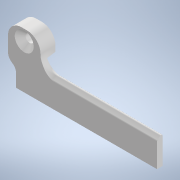
# Autodesk Inventor part: wifi_fixator
Saved by Autodesk Inventor 2022 (Build 260153000, 153)
## iProperties
Created: 2025-01-04
Part Number: wifi_fixator
Material: Типовые
Document SubType Name: Modeling
Designer: akap
Density: 1 g/cm^3
Appearance: По умолчанию
Author: akap
Autodesk Inventor part; units mm, degrees
ref_plane "YZ Plane" through (0, 0, 0) normal (1, 0, 0) x (0, 1, 0)
ref_plane "XZ Plane" through (0, 0, 0) normal (0, 1, 0) x (-1, 0, 0)
ref_plane "XY Plane" through (0, 0, 0) normal (0, 0, 1) x (1, 0, 0)
sketch "Эскиз1" plane through (0, 0, 0) normal (0, 0, 1) x (1, 0, 0)
  line L0 (26, -11.6) -> (-26, -11.6)
  line L1 (-26, -11.6) -> (-26, 11.6)
  line L2 (-26, 11.6) -> (26, 11.6)
  line L3 (26, 11.6) -> (26, -11.6)
  line L4 (-27, -1.6037) -> (27, -1.6037)
  line L5 (27, -8.6037) -> (27, -1.6037)
  line L6 (-27, -8.6037) -> (27, -8.6037)
  line L7 (-27, -1.6037) -> (-27, -8.6037)
  line L8 (-25.5, 7) -> (21, 7)
  arc A0 (23, 5) -> (21, 7) centre (21, 5) ccw
  line L9 (23, 5) -> (23, -5)
  arc A1 (21, -7) -> (23, -5) centre (21, -5) ccw
  line L10 (21, -7) -> (-29, -7)
  arc A2 (-31, -5) -> (-29, -7) centre (-29, -5) ccw
  line L11 (-31, -5) -> (-31, 5)
  arc A3 (-30, 6.7321) -> (-31, 5) centre (-29, 5) ccw
  circle A4 centre (-50, 0.4) radius 1.35
  circle A5 centre (50, 0.4) radius 1.35
  arc A6 (-33.5169, 9.4302) -> (-33.5169, 14.4302) centre (-33.5169, 11.9302) ccw
  line L12 (-33.5169, 9.4302) -> (-38.5969, 9.4302)
  arc A7 (-38.5969, 14.4302) -> (-38.5969, 9.4302) centre (-38.5969, 11.9302) ccw
  line L13 (-38.5969, 14.4302) -> (-33.5169, 14.4302)
  line L14 (-39.1, 22.9302) -> (-31.1, 22.9302)
  arc A8 (-30.1, 21.9302) -> (-31.1, 22.9302) centre (-31.1, 21.9302) ccw
  line L15 (-30.1, 21.9302) -> (-30.1, 18.9302)
  arc A9 (-31.1, 17.9302) -> (-30.1, 18.9302) centre (-31.1, 18.9302) ccw
  line L16 (-31.1, 17.9302) -> (-39.1, 17.9302)
  arc A10 (-40.1, 18.9302) -> (-39.1, 17.9302) centre (-39.1, 18.9302) ccw
  line L17 (-40.1, 18.9302) -> (-40.1, 21.9302)
  arc A11 (-39.1, 22.9302) -> (-40.1, 21.9302) centre (-39.1, 21.9302) ccw
  arc A12 (-8.8, 26.9302) -> (-6.8, 28.9302) centre (-8.8, 28.9302) ccw
  line L18 (-6.8, 28.9302) -> (-6.8, 33.6939)
  arc A13 (-3.8, 36.6939) -> (-6.8, 33.6939) centre (-3.8, 33.6939) ccw
  line L19 (-3.8, 36.6939) -> (15.7, 36.6939)
  arc A14 (18.7, 33.6939) -> (15.7, 36.6939) centre (15.7, 33.6939) ccw
  line L20 (18.7, 33.6939) -> (18.7, 19.9302)
  arc A15 (15.7, 16.9302) -> (18.7, 19.9302) centre (15.7, 19.9302) ccw
  line L21 (15.7, 16.9302) -> (-14.8, 16.9302)
  arc A16 (-16.8, 18.9302) -> (-14.8, 16.9302) centre (-14.8, 18.9302) ccw
  line L22 (-16.8, 18.9302) -> (-16.8, 24.9302)
  arc A17 (-14.8, 26.9302) -> (-16.8, 24.9302) centre (-14.8, 24.9302) ccw
  line L23 (-14.8, 26.9302) -> (-8.8, 26.9302)
  circle A18 centre (23.0046, 15.7286) radius 1.5
  circle A19 centre (-23.0046, 15.7286) radius 1.5
  line L24 (-21.9, 127.8) -> (-29.3, 127.8)
  line L25 (-29.3, 127.8) -> (-29.3, 142.3)
  line L26 (-29.3, 142.3) -> (-21.9, 142.3)
  line L27 (-21.9, 142.3) -> (-21.9, 127.8)
  line L28 (29.3, 127.8) -> (21.9, 127.8)
  line L29 (21.9, 127.8) -> (21.9, 142.3)
  line L30 (21.9, 142.3) -> (29.3, 142.3)
  line L31 (29.3, 142.3) -> (29.3, 127.8)
  line L32 (-17.5, 135.4) -> (-17.5, 146.4)
  line L33 (-52.7636, 146.4) -> (-17.5, 146.4)
  spline S0 degree 4 poles (-62.3095, 142.4) (-60.4837, 144.6746) (-58.1635, 146.0345) (-55.4517, 146.4) (-52.7636, 146.4) knots 0 0 0 0 0 1 1 1 1 1
  spline S1 degree 4 poles (-66.7947, 122.4) (-66.7947, 127.5863) (-66.4694, 134.187) (-64.879, 139.1991) (-62.3095, 142.4) knots 0 0 0 0 0 0.584588 0.584588 0.584588 0.584588 0.584588
  line L34 (-66.7947, 12.4) -> (-66.7947, 122.4)
  spline S2 degree 4 poles (-62.3095, -7.6) (-64.879, -4.3991) (-66.4694, 0.613) (-66.7947, 7.2137) (-66.7947, 12.4) knots 0.415412 0.415412 0.415412 0.415412 0.415412 1 1 1 1 1
  spline S3 degree 4 poles (-52.7636, -11.6) (-55.4517, -11.6) (-58.1635, -11.2345) (-60.4837, -9.8746) (-62.3095, -7.6) knots 0 0 0 0 0 1 1 1 1 1
  line L35 (52.7636, -11.6) -> (-52.7636, -11.6)
  spline S4 degree 4 poles (62.3095, -7.6) (60.4837, -9.8746) (58.1635, -11.2345) (55.4517, -11.6) (52.7636, -11.6) knots 0 0 0 0 0 1 1 1 1 1
  spline S5 degree 4 poles (66.7947, 12.4) (66.7947, 7.2137) (66.4694, 0.613) (64.879, -4.3991) (62.3095, -7.6) knots 0 0 0 0 0 0.584588 0.584588 0.584588 0.584588 0.584588
  line L36 (66.7947, 122.4) -> (66.7947, 12.4)
  spline S6 degree 4 poles (62.3095, 142.4) (64.879, 139.1991) (66.4694, 134.187) (66.7947, 127.5863) (66.7947, 122.4) knots 0.415412 0.415412 0.415412 0.415412 0.415412 1 1 1 1 1
  spline S7 degree 4 poles (52.7636, 146.4) (55.4517, 146.4) (58.1635, 146.0345) (60.4837, 144.6746) (62.3095, 142.4) knots 0 0 0 0 0 1 1 1 1 1
  line L37 (17.5, 146.4) -> (52.7636, 146.4)
  line L38 (17.5, 146.4) -> (17.5, 135.4)
  line L39 (17.5, 135.4) -> (6, 135.4)
  line L40 (6, 135.4) -> (6, 130.5467)
  arc A20 (5, 129.5467) -> (6, 130.5467) centre (5, 130.5467) ccw
  line L41 (5, 129.5467) -> (-5, 129.5467)
  arc A21 (-6, 130.5467) -> (-5, 129.5467) centre (-5, 130.5467) ccw
  line L42 (-6, 130.5467) -> (-6, 135.4)
  line L43 (-6, 135.4) -> (-17.5, 135.4)
  circle A22 centre (-25.5, 37.9) radius 1.25
  circle A23 centre (25.5, 96.9) radius 1.25
  circle A24 centre (-25.5, 96.9) radius 1.25
  circle A25 centre (25.5, 37.9) radius 1.25
  arc A26 (22.1, 92.345) -> (25.1, 89.345) centre (25.1, 92.345) ccw
  line L44 (25.1, 89.345) -> (43.5, 89.345)
  line L45 (43.5, 125.4) -> (43.5, 89.345)
  arc A27 (45.5, 127.4) -> (43.5, 125.4) centre (45.5, 125.4) ccw
  line L46 (45.5, 127.4) -> (60.7947, 127.4)
  arc A28 (62.7947, 125.4) -> (60.7947, 127.4) centre (60.7947, 125.4) ccw
  line L47 (62.7947, 125.4) -> (62.7947, 9.4)
  arc A29 (60.7947, 7.4) -> (62.7947, 9.4) centre (60.7947, 9.4) ccw
  line L48 (60.7947, 7.4) -> (45.5, 7.4)
  arc A30 (43.5, 9.4) -> (45.5, 7.4) centre (45.5, 9.4) ccw
  line L49 (43.5, 45.3296) -> (43.5, 9.4)
  line L50 (43.5, 45.3296) -> (27.6138, 45.3296)
  line L51 (27.6138, 45.3296) -> (27.6138, 44.2037)
  line L52 (27.6138, 44.2037) -> (10.238, 44.2037)
  line L53 (10.238, 44.2037) -> (10.238, 45.3296)
  line L54 (10.238, 45.3296) -> (5, 45.3296)
  line L55 (5, 45.3296) -> (5, 42.3296)
  line L56 (5, 42.3296) -> (-5, 42.3296)
  line L57 (-5, 42.3296) -> (-5, 45.3296)
  line L58 (-5, 45.3296) -> (-10.238, 45.3296)
  line L59 (-10.238, 45.3296) -> (-10.238, 44.2037)
  line L60 (-10.238, 44.2037) -> (-27.6138, 44.2037)
  line L61 (-27.6138, 44.2037) -> (-27.6138, 45.3296)
  line L62 (-27.6138, 45.3296) -> (-29.6, 45.3296)
  line L63 (-29.6, 45.3296) -> (-29.6, 27.7796)
  line L64 (-29.6, 27.7796) -> (-40.6, 27.7796)
  line L65 (-40.6, 27.7796) -> (-40.6, 45.3296)
  line L66 (-40.6, 45.3296) -> (-43.5, 45.3296)
  line L67 (-43.5, 9.4) -> (-43.5, 45.3296)
  arc A31 (-45.5, 7.4) -> (-43.5, 9.4) centre (-45.5, 9.4) ccw
  line L68 (-45.5, 7.4) -> (-60.7947, 7.4)
  arc A32 (-62.7947, 9.4) -> (-60.7947, 7.4) centre (-60.7947, 9.4) ccw
  line L69 (-62.7947, 9.4) -> (-62.7947, 125.4)
  arc A33 (-60.7947, 127.4) -> (-62.7947, 125.4) centre (-60.7947, 125.4) ccw
  line L70 (-60.7947, 127.4) -> (-45.5, 127.4)
  arc A34 (-43.5, 125.4) -> (-45.5, 127.4) centre (-45.5, 125.4) ccw
  line L71 (-43.5, 89.345) -> (-43.5, 125.4)
  line L72 (-43.5, 89.345) -> (-40.6, 89.345)
  line L73 (-40.6, 89.345) -> (-40.6, 104.345)
  line L74 (-40.6, 104.345) -> (-28.1, 104.345)
  line L75 (-28.1, 104.345) -> (-28.1, 89.345)
  line L76 (-28.1, 89.345) -> (-18.1, 89.345)
  arc A35 (-18.1, 89.345) -> (-15.1, 92.345) centre (-18.1, 92.345) ccw
  line L77 (-15.1, 92.345) -> (-15.1, 99.8467)
  arc A36 (-12.1, 102.8467) -> (-15.1, 99.8467) centre (-12.1, 99.8467) ccw
  line L78 (-12.1, 102.8467) -> (19.1, 102.8467)
  arc A37 (22.1, 99.8467) -> (19.1, 102.8467) centre (19.1, 99.8467) ccw
  line L79 (22.1, 99.8467) -> (22.1, 92.345)
  line L80 (28, -0.6037) -> (-28, -0.6037)
  line L81 (-28, -0.6037) -> (-28, -9.6037)
  line L82 (-28, -9.6037) -> (28, -9.6037)
  line L83 (28, -9.6037) -> (28, -0.6037)
  line L84 (-40.5, 5.2533) -> (-27, 5.2533)
  line L85 (-27, 5.2533) -> (-27, -1.6037)
  line L86 (-26, -1.6037) -> (-26, 6.2533)
  line L87 (-26, 6.2533) -> (-40.5, 6.2533)
  line L88 (-26, 6.2533) -> (-29, 6.2533)
  line L89 (-29, 6.2533) -> (-29, 19.7286)
  line L90 (-29, 19.7286) -> (-17, 19.7286)
  line L91 (-17, 19.7286) -> (-17, 7)
  line L92 (-26, -1.6037) -> (27, -1.6037)
  line L93 (27, -1.6037) -> (27, 7)
  line L94 (27, 7) -> (-26, 7)
  line L95 (-26, 7) -> (-26, -1.6037)
  arc A38 (-30, 6.7321) -> (-29.5, 7.5981) centre (-30.5, 7.5981) ccw
  line L96 (-29.5, 7.5981) -> (-29.5, 12.6)
  line L97 (-29.5, 12.6) -> (-26.5, 12.6)
  line L98 (-26.5, 12.6) -> (-26.5, 8)
  arc A39 (-26.5, 8) -> (-25.5, 7) centre (-25.5, 8) ccw
  point P0 (0, 0)
  point P1 (26, -0.6037)
  point P2 (-17, 11.6)
  point P3 (-29, 7)
  point P4 (-26, 7)
  point P5 (-26, -0.6037)
  point P6 (23, -0.6037)
  point P7 (-26, -7)
  point P8 (-29, 12.6)
  point P9 (-26, 7.134)
  dimension "d0" = 1
  dimension "d1" = 1
  dimension "d2" = 3
  dimension "d3" = 4
  dimension "d4" = 12
  constraints: 28 end point, 3 collinear, 3 perpendicular, 2 parallel, 2 point on line, 1 horizontal, 1 vertical, 4 other
  measures "d0" distance between parallel lines of L4 L80
  measures "d1" distance between parallel lines of L85 L86
  measures "d2" distance of L86.end L88.end
  measures "d3" distance from line of L90 A19.centre
  measures "d4" distance between parallel lines of L89 L91
extrude "Выдавливание1" add sketch "Эскиз1" along normal blind 2 contours L80 L9 A0 L94 L3 | L94 L8 L91 L2 L3 | L80 L1 L94 L8 A0 L9 | L87 L89 L97 L98 A39 L1 | L91 L8 A39 L1 L2 | L2 L1 A39 L98 L97 L89 L90 L91 | L1 A39 L94
sketch "Эскиз2" plane through (0, 0, 0) normal (0, 0, -1) x (-1, 0, 0)
  line L0 (-26, -0.6037) -> (-26, 11.6) projected
  line L1 (-26, 11.6) -> (17, 11.6) projected
  line L2 (17, 11.6) -> (17, 19.7286) projected
  line L3 (17, 19.7286) -> (29, 19.7286) projected
  line L4 (29, 19.7286) -> (29, 6.2533) projected
  line L5 (26, 6.2533) -> (26, -0.6037) projected
  line L6 (26, -0.6037) -> (-26, -0.6037) projected
  line L7 (-26, -11.6) -> (26, -11.6) projected
  line L8 (-26, 11.6) -> (-26, -11.6) projected
  line L9 (26, 11.6) -> (-26, 11.6) projected
  line L10 (26, -11.6) -> (26, 11.6) projected
  line L11 (-27, 12.6) -> (-27, -12.6)
  line L12 (-27, -12.6) -> (27, -12.6)
  line L13 (27, -12.6) -> (27, 12.6)
  line L14 (27, 12.6) -> (-27, 12.6)
  line L15 (29, 6.2533) -> (26, 6.2533) projected
  circle A0 centre (23.0046, 15.7286) radius 1.5 projected
  point P0 (0, 0)
  point P1 (26, 7)
  point P2 (17, 12.6)
  point P3 (27, 6.2533)
  dimension "d7" = 1
  constraints: 8 end point, 3 other
  measures "d7" distance between parallel lines of L9 L14
extrude "Выдавливание2" add sketch "Эскиз2" along normal blind 3.5 contours L2 L3 L4 L15 L13 L14
fillet "Сопряжение1" radius 5 2 edges at (-17, 19.7286, -0.75) (-29, 19.7286, -0.75)
chamfer "Фаска1" distance 2 angle 45 1 edges at (-24.5046, 15.7286, 2)
sketch "Эскиз3" plane through (26, -0.6037, 0) normal (1, 0, 0) x (0, 0, -1)
  circle A0 centre (-10.5, 18.857) radius 13 projected
  point P0 (0, 0.6037)
extrude "Выдавливание3" cut sketch "Эскиз3" against normal up to surface (43 mm away)
fillet "Сопряжение2" radius 0.5 2 edges at (4.5, 10.5884, 0) (4.5, 8.4171, 2)
fillet "Сопряжение3" radius 3 2 edges at (-26, 6.2533, 1) (-29, 6.2533, -0.75)
fillet "Сопряжение4" radius 5 3 edges at (-17, 8.3951, 1.9564) (-17, 9.6505, 0.32) (-17, 9.0292, 1.3394)
fillet "Сопряжение5" radius 0.8 1 edges at (-27, 6.2932, -1.75)
